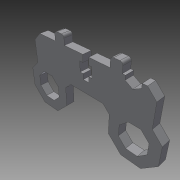
# Autodesk Inventor part: filament_guide
Saved by Autodesk Inventor 2014 (Build 180170000, 170)
## iProperties
Created: 2014-04-16
Part Number: filament_guide
Material: Plywood, Finish
Document SubType Name: Modeling
Designer: buben
Density: 0.552 g/cm^3
Appearance: Plywood - New
Author: buben
Autodesk Inventor part; units mm, degrees
ref_plane "YZ Plane" through (0, 0, 0) normal (1, 0, 0) x (0, 1, 0)
ref_plane "XZ Plane" through (0, 0, 0) normal (0, 1, 0) x (-1, 0, 0)
ref_plane "XY Plane" through (0, 0, 0) normal (0, 0, 1) x (1, 0, 0)
sketch "Sketch1" plane through (0, 0, 0) normal (0, 1, 0) x (-1, 0, 0)
  line L0 (0, 0) -> (-81, 0)
  line L1 (6, -23.0013) -> (13, -30.0013)
  line L2 (13, -30.0013) -> (13, -44.4987)
  line L3 (13, -44.4987) -> (2.7487, -54.75)
  line L4 (2.7487, -54.75) -> (-11.7487, -54.75)
  line L5 (-11.7487, -54.75) -> (-22, -44.4987)
  line L6 (-22, -44.4987) -> (-22, -30.0013)
  line L7 (-59, -30.0013) -> (-59, -44.4987)
  line L8 (-59, -44.4987) -> (-69.2513, -54.75)
  line L9 (-69.2513, -54.75) -> (-83.7487, -54.75)
  line L10 (-83.7487, -54.75) -> (-94, -44.4987)
  line L11 (-94, -44.4987) -> (-94, -30.0013)
  line L12 (-94, -30.0013) -> (-87, -23.0013)
  line L13 (-4.5, -37.25) -> (-76.5, -37.25) construction
  line L14 (-8.6421, -27.25) -> (-0.3579, -27.25)
  line L15 (-0.3579, -27.25) -> (5.5, -33.1079)
  line L16 (5.5, -33.1079) -> (5.5, -41.3921)
  line L17 (5.5, -41.3921) -> (-0.3579, -47.25)
  line L18 (-0.3579, -47.25) -> (-8.6421, -47.25)
  line L19 (-8.6421, -47.25) -> (-14.5, -41.3921)
  line L20 (-14.5, -41.3921) -> (-14.5, -33.1079)
  line L21 (-14.5, -33.1079) -> (-8.6421, -27.25)
  line L22 (-80.6421, -27.25) -> (-72.3579, -27.25)
  line L23 (-72.3579, -27.25) -> (-66.5, -33.1079)
  line L24 (-66.5, -33.1079) -> (-66.5, -41.3921)
  line L25 (-66.5, -41.3921) -> (-72.3579, -47.25)
  line L26 (-72.3579, -47.25) -> (-80.6421, -47.25)
  line L27 (-80.6421, -47.25) -> (-86.5, -41.3921)
  line L28 (-86.5, -41.3921) -> (-86.5, -33.1079)
  line L29 (-86.5, -33.1079) -> (-80.6421, -27.25)
  line L30 (6, -23.0013) -> (6, -6)
  line L31 (6, -6) -> (0, 0)
  line L32 (-81, 0) -> (-87, -6)
  line L33 (-87, -6) -> (-87, -23.0013)
  line L34 (-22, -30.0013) -> (-27.0013, -25)
  line L35 (-27.0013, -25) -> (-53.9987, -25)
  line L36 (-53.9987, -25) -> (-59, -30.0013)
  point P0 (-40.5, -37.25)
  point P1 (-40.5, 0)
  dimension "d0" = 81
  dimension "d1" = 37.25
  dimension "d2" = 72
  dimension "d3" = 20
  dimension "d4" = 20
  dimension "d5" = 45
  dimension "d6" = 6
  dimension "d7" = 35
  dimension "d8" = 35
  dimension "d17" = 7
  dimension "d20" = 45
  dimension "d21" = 25
  constraints: 74 end point, 5 perpendicular, 3 horizontal, 2 coincident, 2 midpoint, 2 parallel, 1 horizontal alignment, 1 vertical alignment, 56 other
  measures "d0" distance of L0.start L0.end
  measures "d1" distance from line of L13.start L0
  measures "d2" distance of L13.end L13.start
  measures "d3" distance between parallel lines of L20 L16
  measures "d4" distance between parallel lines of L28 L24
  measures "d5" angle of L0 L31
  measures "d6" horizontal distance of L30.end L0.start
  measures "d7" distance between parallel lines of L6 L2
  measures "d8" distance between parallel lines of L11 L7
  measures "d17" distance between parallel lines of L2 L30
  measures "d20" angle of L6 L34
  measures "d21" distance between parallel lines of L0 L35
extrude "Extrusion1" add sketch "Sketch1" along normal blind 6.5
sketch "Sketch2" plane through (0, 6.5, 0) normal (0, 1, 0) x (1, 0, 0)
  line L0 (0, 0) -> (81, 0) projected
  line L1 (38.25, 16.3) -> (42.75, 16.3)
  line L2 (42.75, 0) -> (38.25, 0)
  line L3 (45.25, 12.3) -> (45.25, 5)
  line L4 (35.75, 5) -> (35.75, 12.3)
  line L5 (38.25, 0) -> (38.25, 5)
  line L6 (38.25, 12.3) -> (38.25, 16.3)
  line L7 (42.75, 16.3) -> (42.75, 12.3)
  line L8 (42.75, 5) -> (42.75, 0)
  line L9 (35.75, 12.3) -> (38.25, 12.3)
  line L10 (42.75, 12.3) -> (45.25, 12.3)
  line L11 (45.25, 5) -> (42.75, 5)
  line L12 (38.25, 5) -> (35.75, 5)
  point P0 (40.5, 0)
  dimension "d24" = 4.5
  dimension "d25" = 4
  dimension "d26" = 5
  dimension "d27" = 7.3
  dimension "d28" = 2.5
  constraints: 24 end point, 10 parallel, 5 collinear, 4 perpendicular, 3 horizontal, 2 midpoint
  measures "d24" distance of L1.start L1.end
  measures "d25" distance of L1.end L7.end
  measures "d26" distance of L8.start L2.start
  measures "d27" distance of L3.start L3.end
  measures "d28" distance of L4.end L6.start
extrude "Extrusion2" cut sketch "Sketch2" against normal through all
sketch "Sketch3" plane through (0, 6.5, 0) normal (0, 1, 0) x (1, 0, 0)
  line L0 (42.75, 0) -> (81, 0) projected
  line L1 (0, 0) -> (38.25, 0) projected
  line L2 (38.25, 16.3) -> (42.75, 16.3) projected
  line L3 (15, 0) -> (23, 0)
  line L4 (23, 0) -> (23, -4.5)
  line L5 (21, -6.5) -> (17, -6.5)
  line L6 (15, -4.5) -> (15, 0)
  line L7 (58, 0) -> (66, 0)
  line L8 (66, 0) -> (66, -4.5)
  line L9 (64, -6.5) -> (60, -6.5)
  line L10 (58, -4.5) -> (58, 0)
  arc A0 (15, -4.5) -> (17, -6.5) centre (17, -4.5) ccw
  arc A1 (21, -6.5) -> (23, -4.5) centre (21, -4.5) ccw
  arc A2 (58, -4.5) -> (60, -6.5) centre (60, -4.5) ccw
  arc A3 (64, -6.5) -> (66, -4.5) centre (64, -4.5) ccw
  point P0 (40.5, 16.3)
  dimension "d31" = 2
  dimension "d32" = 8
  dimension "d33" = 8
  dimension "d34" = 6.5
  dimension "d35" = 35
  dimension "d36" = 17.5
  constraints: 16 end point, 8 point on circle, 8 tangent, 4 centre point, 4 parallel, 3 equal radius, 2 horizontal, 2 perpendicular, 2 point on line, 1 collinear, 1 midpoint
  measures "d31" radius of A0
  measures "d32" distance between parallel lines of L8 L10
  measures "d33" distance between parallel lines of L6 L4
  measures "d34" distance between parallel lines of L3 L5
  measures "d35" distance between parallel lines of L10 L4
  measures "d36" distance from line of point (40.5, 16.3) L4
extrude "Extrusion3" add sketch "Sketch3" against normal blind 6.5
sketch "Sketch4" plane through (0, 6.5, 0) normal (0, 1, 0) x (1, 0, 0)
  line L0 (66, -4.5) -> (66, 0) projected
  line L1 (66, 0) -> (81, 0) projected
  line L2 (73, 5.7735) -> (78, 2.8868)
  line L3 (78, 2.8868) -> (78, 0)
  line L4 (68, 0) -> (68, 2.8868)
  line L5 (68, 2.8868) -> (73, 5.7735)
  line L6 (78, 0) -> (68, 0)
  point P0 (73, 0)
  dimension "d39" = 10
  dimension "d40" = 2
  constraints: 10 end point, 3 point on line, 1 collinear, 1 horizontal alignment, 6 other
  measures "d39" distance between parallel lines of L4 L3
  measures "d40" distance between parallel lines of L0 L4
extrude "Extrusion4" cut sketch "Sketch4" against normal through all
equation "\"d33\" = d32"
equation "\"d36\" = 0.5 * d35"
body "Solid1"
